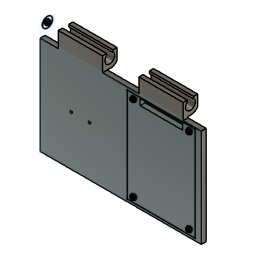
case-screen (Autodesk Fusion 360 design; units mm, degrees)
Autodesk Fusion 360 part; units mm, degrees
sketch "Esboço1" plane through (0, 0, 0) normal (0, 1, 0) x (1, 0, 0)
  line L0 (33.25, -20.5) -> (-33.25, -20.5)
  line L1 (-33.25, -20.5) -> (-33.25, 20.5)
  line L2 (-33.25, 20.5) -> (33.25, 20.5)
  line L3 (33.25, 20.5) -> (33.25, -20.5)
  dimension "d1" = 66.5
  dimension "d2" = 41
  dimension "d3" = 20.5
  dimension "d4" = 33.25
  constraint horizontal L0
  constraint vertical L1
  constraint horizontal L2
  constraint vertical L3
  measures "d1" distance of L0.start L0.end
  measures "d2" distance of L0.start L2.end
  measures "d3" distance of origin L0
  measures "d4" distance of origin L3
extrude "Extrusão1" add sketch "Esboço1" along normal blind 2
sketch "Esboço2" plane through (0, 0, 0) normal (0, -1, 0) x (1, 0, 0)
  line L0 (-33.25, -20.5) -> (33.25, -20.5)
  line L1 (33.25, -20.5) -> (33.25, 20.5)
  line L2 (33.25, 20.5) -> (-33.25, 20.5)
  line L3 (-33.25, 20.5) -> (-33.25, -20.5)
  line L4 (30.75, 19.5) -> (2.75, 19.5)
  line L5 (2.75, 19.5) -> (2.75, -19.5)
  line L6 (2.75, -19.5) -> (30.75, -19.5)
  line L7 (30.75, -19.5) -> (30.75, 19.5)
  circle A0 centre (28.25, -17.5) radius 1
  circle A1 centre (5.25, -17.5) radius 1
  circle A2 centre (5.25, 17.5) radius 1
  circle A3 centre (28.25, 17.5) radius 1
  point P0 (28.25, 17.5)
  point P1 (5.25, 17.5)
  point P2 (28.25, -17.5)
  point P3 (5.25, -17.5)
  dimension "d7" = 28
  dimension "d8" = 39
  dimension "d9" = 1
  dimension "d10" = 2.5
  dimension "d11" = 2
  dimension "d12" = 2.5
  dimension "d13" = 2.5
  dimension "d14" = 2
  dimension "d15" = 2
  dimension "d16" = 2.5
  dimension "d17" = 2.5
  dimension "d18" = 2
  dimension "d19" = 2
  dimension "d20" = 2
  dimension "d21" = 2
  dimension "d22" = 2
  constraint horizontal L4
  constraint vertical L5
  constraint horizontal L6
  constraint vertical L7
  constraint coincident P2 A0.centre
  constraint coincident P3 A1.centre
  constraint coincident P1 A2.centre
  constraint coincident P0 A3.centre
  measures "d7" distance of L4.start L4.end
  measures "d8" distance of L4.start L6.end
  measures "d9" distance of L2 L4
  measures "d10" distance of L1 L7
  measures "d11" distance of L4 P0
  measures "d12" distance of L7 P0
  measures "d13" distance of L5 P1
  measures "d14" distance of L4 P1
  measures "d15" distance of L6 P3
  measures "d16" distance of L5 P3
  measures "d17" distance of L7 P2
  measures "d18" distance of L6 P2
  measures "d19" diameter of A0
  measures "d20" diameter of A1
  measures "d21" diameter of A2
  measures "d22" diameter of A3
hole "Furo1" at (5.25, 0, 17.5) at (28.25, 0, 17.5) at (28.25, 0, -17.5) at (5.25, 0, -17.5) direction (0, 1, 0) diameter 2 depth 6 tip angle 118
sketch "Esboço3" plane through (0, 0, 0) normal (0, -1, 0) x (1, 0, 0)
  circle A0 centre (28.25, -17.5) radius 1
  circle A1 centre (5.25, 17.5) radius 1
  circle A2 centre (28.25, 17.5) radius 1
  circle A3 centre (5.25, -17.5) radius 1
  line L0 (-33.25, -20.5) -> (33.25, -20.5)
  line L1 (33.25, -20.5) -> (33.25, 20.5)
  line L2 (33.25, 20.5) -> (-33.25, 20.5)
  line L3 (-33.25, 20.5) -> (-33.25, -20.5)
  line L4 (8, 19) -> (25.5, 19)
  line L5 (25.5, 19) -> (25.5, 16.5)
  line L6 (25.5, 16.5) -> (8, 16.5)
  line L7 (8, 16.5) -> (8, 19)
  line L8 (30.75, -19.5) -> (30.75, 19.5)
  line L9 (30.75, 19.5) -> (2.75, 19.5)
  dimension "d26" = 17.5
  dimension "d27" = 2.5
  dimension "d28" = 5.25
  dimension "d29" = 0.5
  constraint horizontal L4
  constraint vertical L5
  constraint horizontal L6
  constraint vertical L7
  measures "d26" distance of L4.start L4.end
  measures "d27" distance of L4.start L6.end
  measures "d28" distance of L5 L8
  measures "d29" distance of L4 L9
extrude "Extrusão2" cut sketch "Esboço3" against normal blind 2 contours L4 L5 L6 L7
sketch "Esboço4" plane through (0, 0, 0) normal (0, -1, 0) x (1, 0, 0)
  circle A0 centre (-16.625, 0) radius 5.875
  point P0 (-20.375, 0)
  point P1 (-12.875, 0)
  dimension "d32" = 11.75
  dimension "d33" = 16.625
  dimension "d34" = 7.5
  dimension "d35" = 3.75
  measures "d32" diameter of A0
  measures "d33" distance of origin A0.centre
  measures "d34" distance of P0 P1
  measures "d35" distance of A0.centre P1
hole "Furo2" at (-20.375, 0, 0) at (-12.875, 0, 0) direction (0, 1, 0) diameter 1 depth 6 tip angle 118
sketch "Esboço5" plane through (0, 0, 20.5) normal (0, 0, 1) x (-1, 0, 0)
  line L0 (33.25, 0) -> (-33.25, 0)
  line L1 (-33.25, 0) -> (-33.25, -2)
  line L2 (-33.25, -2) -> (33.25, -2)
  line L3 (33.25, -2) -> (33.25, 0)
  line L4 (-33.25, 0) -> (33.25, 0)
  line L5 (33.25, 0) -> (33.25, -6)
  line L6 (33.25, -6) -> (-33.25, -6)
  line L7 (-33.25, -6) -> (-33.25, 0)
  dimension "d39" = 66.5
  dimension "d40" = 6
  constraint horizontal L4
  constraint vertical L5
  constraint horizontal L6
  constraint vertical L7
  constraint coincident L0.end L1.start
  measures "d39" distance of L0.end L0.start
  measures "d40" distance of L0.end L6.end
extrude "Extrusão3" add sketch "Esboço5" along normal blind 5
sketch "Esboço6" plane through (-33.25, 0, 0) normal (-1, 0, 0) x (0, -1, 0)
  line L0 (0, -20.5) -> (0, 25.5)
  line L1 (0, 25.5) -> (-6, 25.5)
  line L2 (-6, 25.5) -> (-6, 20.5)
  line L3 (-6, 20.5) -> (-2, 20.5)
  line L4 (-2, 20.5) -> (-2, -20.5)
  line L5 (-2, -20.5) -> (0, -20.5)
  circle A0 centre (-3, 24.2) radius 2.05
  point P0 (-3, 24.2)
  dimension "d43" = 3
  dimension "d44" = 1.3
  dimension "d45" = 4.1
  constraint coincident P0 A0.centre
  measures "d43" distance of L2 P0
  measures "d44" distance of L1 P0
  measures "d45" diameter of A0
extrude "Extrusão4" cut sketch "Esboço6" against normal blind 70 contours L1 A0 picked at (-2.4423, 23.4445)
sketch "Esboço7" plane through (-33.25, 0, 0) normal (-1, 0, 0) x (0, -1, 0)
  arc A0 (-4.5851, 25.5) -> (-1.4149, 25.5) centre (-3, 24.2) ccw
  line L0 (-4.5851, 25.5) -> (-6, 25.5)
  line L1 (-6, 25.5) -> (-6, 20.5)
  line L2 (-6, 20.5) -> (-2, 20.5)
  line L3 (-2, 20.5) -> (-2, -20.5)
  line L4 (-2, -20.5) -> (0, -20.5)
  line L5 (0, -20.5) -> (0, 25.5)
  line L6 (0, 25.5) -> (-1.4149, 25.5)
  circle A1 centre (-3, 24.2) radius 2.5
  circle A2 centre (-3, 24.2) radius 3.8
  line L7 (-6, 21.8676) -> (-6, 20.5)
  dimension "d48" = 5
  dimension "d57" = 7.6
  constraint concentric A0 A1
  constraint concentric A1 A2
  constraint coincident A2 L7.start
  constraint coincident L1 L7.start
  constraint coincident L1.end L2.start
  measures "d48" diameter of A1
  measures "d57" diameter of A2
extrude "Extrusão5" cut sketch "Esboço7" against normal blind 70 contours L1 L2 A2 L7
sketch "Esboço8" plane through (0, 0, 0) normal (0, -1, 0) x (1, 0, 0)
  line L0 (33.25, -20.5) -> (33.25, 25.5)
  line L1 (33.25, 25.5) -> (-33.25, 25.5)
  line L2 (-33.25, 25.5) -> (-33.25, -20.5)
  line L3 (-7.5, 25.5) -> (7.5, 25.5)
  line L4 (7.5, 25.5) -> (7.5, 20.5)
  line L5 (7.5, 20.5) -> (-7.5, 20.5)
  line L6 (-7.5, 20.5) -> (-7.5, 25.5)
  line L7 (-33.25, 25.5) -> (-25.75, 25.5)
  line L8 (-25.75, 25.5) -> (-25.75, 20)
  line L9 (-25.75, 20) -> (-33.25, 20)
  line L10 (-33.25, 20) -> (-33.25, 25.5)
  line L11 (0, 1.75) -> (0, 22.5)
  line L12 (33.25, 20) -> (33.25, 25.5)
  line L13 (25.75, 25.5) -> (25.75, 20)
  line L14 (25.75, 20) -> (33.25, 20)
  line L15 (33.25, 25.5) -> (25.75, 25.5)
  circle A0 centre (-20.375, 0) radius 0.5
  circle A1 centre (-12.875, 0) radius 0.5
  line L16 (25.5, 19) -> (25.5, 16.5)
  line L17 (25.5, 16.5) -> (8, 16.5)
  line L18 (8, 16.5) -> (8, 19)
  line L19 (8, 19) -> (25.5, 19)
  circle A2 centre (28.25, -17.5) radius 1
  circle A3 centre (5.25, 17.5) radius 1
  circle A4 centre (28.25, 17.5) radius 1
  circle A5 centre (5.25, -17.5) radius 1
  line L20 (-33.25, -20.5) -> (33.25, -20.5)
  point P0 (33.25, 25.5)
  dimension "d51" = 15
  dimension "d52" = 5
  dimension "d53" = 25.75
  dimension "d56" = 7.5
  constraint horizontal L3
  constraint vertical L4
  constraint horizontal L5
  constraint vertical L6
  constraint coincident L1 L3.start
  constraint horizontal L7
  constraint vertical L8
  constraint horizontal L9
  constraint vertical L10
  constraint coincident L1.end L2.start
  constraint symmetric L1.end L11 P0
  constraint symmetric L7.end L11 L13.start
  constraint symmetric L8.end L11 L13.end
  constraint symmetric L9.end L11 L12.start
  measures "d51" distance of L3.start L3.end
  measures "d52" distance of L3.start L5.end
  measures "d53" distance of L0 L4
  measures "d56" distance of L1.end L7.end
extrude "Extrusão6" cut sketch "Esboço8" against normal blind 10 contours L0 L1 L12 L13 L14 L15 | L1 L2 L7 L8 L9 L10 | L1 L3 L4 L5 L6
extrude "Extrusão7" add 4 faces at (19.6667, 0.4716, 25.5) (-13.5833, 0.4716, 25.5) (-13.5833, 5.0567, 25.5) (19.6667, 5.5284, 25.5) along direction (0, 0, 1) blind 1
sketch "Esboço9" plane through (0, 2, 0) normal (0, 1, 0) x (-1, 0, 0)
  line L0 (25.75, 20) -> (25.75, 20.5)
  line L1 (25.75, 20.5) -> (7.5, 20.5)
  line L2 (-25.75, 20.5) -> (-25.75, 20)
  line L3 (-25.75, 20) -> (-33.25, 20)
  line L4 (-33.25, 20) -> (-33.25, -20.5)
  line L5 (-33.25, -20.5) -> (33.25, -20.5)
  line L6 (33.25, -20.5) -> (33.25, 20)
  line L7 (33.25, 20) -> (25.75, 20)
  circle A0 centre (20.375, 0) radius 0.5
  circle A1 centre (12.875, 0) radius 0.5
  line L8 (-25.5, 16.5) -> (-25.5, 19)
  line L9 (-25.5, 19) -> (-8, 19)
  line L10 (-8, 19) -> (-8, 16.5)
  line L11 (-8, 16.5) -> (-25.5, 16.5)
  circle A2 centre (-28.25, -17.5) radius 1
  circle A3 centre (-5.25, 17.5) radius 1
  circle A4 centre (-28.25, 17.5) radius 1
  circle A5 centre (-5.25, -17.5) radius 1
  line L12 (33.25, -20.5) -> (-40, -20.5)
  line L13 (-40, -20.5) -> (-40, 10)
  line L14 (-40, 10) -> (33.25, 10)
  line L15 (33.25, 10) -> (33.25, -20.5)
  line L16 (7.5, 20.5) -> (-7.5, 20.5)
  line L17 (-7.5, 20.5) -> (-25.75, 20.5)
  constraint horizontal L12
  constraint vertical L13
  constraint horizontal L14
  constraint vertical L15
  constraint coincident L5.end L6.start
extrude "Extrusão8" [suppressed]
extrude "Extrusão9" add 2 faces at (-19.6667, 1.4149, 25.8333) (13.5833, 1.4149, 25.8333) along direction (0, 1, 0) blind 0.25
extrude "Extrusão10" add 2 faces at (13.5833, 4.5851, 25.8333) (-19.6667, 4.5851, 25.8333) along direction (0, -1, 0) blind 0.25
equation "d3 = ( 41 / 2 ) * 1 mm"
equation "d4 = ( 66.5 / 2 ) * 1 mm"
equation "d28 = ( ( 28 - 17.5 ) / 2 ) * 1 mm"
equation "d33 = ( 33.25 / 2 ) * 1 mm"
equation "d35 = ( 7.5 / 2 ) * 1 mm"
equation "d53 = ( ( 66.5 - 15 ) / 2 ) * 1 mm"
